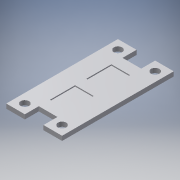
# Autodesk Inventor part: FoldLink
Saved by Autodesk Inventor 2016 (Build 200138000, 138)
## iProperties
Created: 2015-03-29
Part Number: FoldLink
Material: Rubber, Silicone
Document SubType Name: Modeling
Designer: Erin
Density: 1.25 g/cm^3
Appearance: Rubber - Blue - Version 1.1
Mass: 1.17173 g
Surface Area: 20.6631 cm^2
Volume: 0.937383 cm^3
Author: Erin
Autodesk Inventor part; units mm, degrees
ref_plane "YZ Plane" through (0, 0, 0) normal (1, 0, 0) x (0, 1, 0)
ref_plane "XZ Plane" through (0, 0, 0) normal (0, 1, 0) x (-1, 0, 0)
ref_plane "XY Plane" through (0, 0, 0) normal (0, 0, 1) x (1, 0, 0)
sketch "Sketch1" plane through (0, 0, 0) normal (0, 0, 1) x (1, 0, 0)
  line L0 (0, 35.9415) -> (0, -22.75) construction
  line L1 (5, 30) -> (15, 30)
  line L2 (15, 30) -> (15, -30)
  line L3 (15, -30) -> (5, -30)
  line L4 (5, -30) -> (5, 30)
  circle A0 centre (10, 25) radius 2.25
  circle A1 centre (10, -25) radius 2.25
  line L5 (-5, 22.5) -> (5, 22.5)
  line L6 (5, 22.5) -> (5, -22.5)
  line L7 (5, -22.5) -> (-5, -22.5)
  line L8 (-5, -22.5) -> (-5, 22.5)
  line L9 (-5, 22.5) -> (5, 22.5)
  line L10 (5, 22.5) -> (5, 16.5)
  line L11 (5, 16.5) -> (-5, 16.5)
  line L12 (-5, 16.5) -> (-5, 22.5)
  line L13 (-5, -22.5) -> (5, -22.5)
  line L14 (5, -22.5) -> (5, -16.5)
  line L15 (5, -16.5) -> (-5, -16.5)
  line L16 (-5, -16.5) -> (-5, -22.5)
  line L17 (-5, 3) -> (5, 3)
  line L18 (5, 3) -> (5, -3)
  line L19 (5, -3) -> (-5, -3)
  line L20 (-5, -3) -> (-5, 3)
  point P0 (0, 0)
  point P1 (15, 0)
  point P2 (5, 0)
  point P3 (0, 22.5)
  point P4 (5, 0)
  point P5 (5, 0)
  dimension "d28" = 60
  dimension "d29" = 4.5
  dimension "d30" = 4.5
  dimension "d31" = 5
  dimension "d32" = 5
  dimension "d33" = 10
  dimension "d36" = 10
  dimension "d37" = 45
  dimension "d38" = 5
  dimension "d39" = 5
  dimension "d42" = 6
  dimension "d43" = 6
  dimension "d44" = 6
  constraints: 42 end point, 10 parallel, 5 horizontal, 5 midpoint, 5 perpendicular, 3 point on line, 2 centre point, 2 collinear, 2 horizontal alignment, 2 vertical alignment, 1 coincident, 1 vertical
  measures "d28" distance of L1.end L2.end
  measures "d29" diameter of A0
  measures "d30" diameter of A1
  measures "d31" distance from line of A0.centre L1
  measures "d32" distance from line of A0.centre L2
  measures "d33" distance of L1.start L1.end
  measures "d36" distance of L6.end L7.end
  measures "d37" distance of L5.end L6.end
  measures "d38" distance from line of A1.centre L3
  measures "d39" distance from line of A1.centre L2
  measures "d42" distance of L9.end L10.end
  measures "d43" distance of L14.end L13.end
  measures "d44" distance of L17.end L18.end
extrude "Extrusion3" add sketch "Sketch1" along normal blind 1.8 contours L4 L11 L8 L5 | L4 L17 L8 L11 | L4 L19 L8 L17 | L7 L8 L15 L4 | L4 L15 L8 L19
extrude "Extrusion5" add sketch "Sketch1" along normal blind 2.4 contours L1 L2 L3 L4
extrude "Extrusion6" add sketch "Sketch1" along normal blind 2.4 contours L4 L11 L8 L5 | L4 L19 L8 L17 | L7 L8 L15 L4
mirror "Mirror2" about plane through (0, 0, 0) normal (1, 0, 0) of "Extrusion5", "Extrusion6"
equation "\"d29\" = screw"
equation "\"d30\" = screw"
equation "\"screw\" = 4.5"
body "Solid2"
